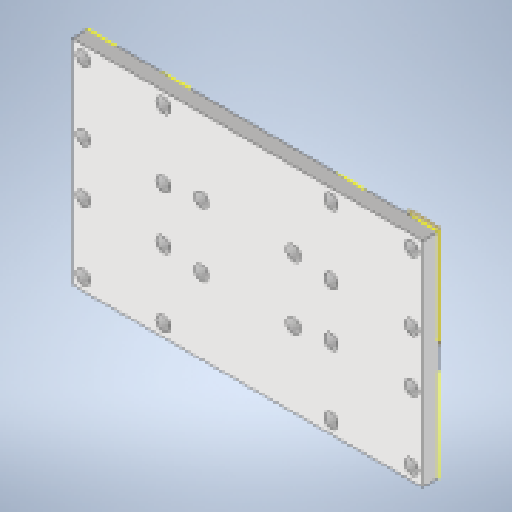
# Autodesk Inventor part: X_PLATE
Saved by Autodesk Inventor 2025.2 (Build 292293000, 293)
## iProperties
Created: 2026-02-06
Part Number: X_PLATE
Material: Generic
Document SubType Name: Modeling
Designer: composite
Density: 1 g/cm^3
Appearance: Default
Author: composite
Autodesk Inventor part; units mm, degrees
ref_plane "YZ Plane" through (0, 0, 0) normal (1, 0, 0) x (0, 1, 0)
ref_plane "XZ Plane" through (0, 0, 0) normal (0, 1, 0) x (-1, 0, 0)
ref_plane "XY Plane" through (0, 0, 0) normal (0, 0, 1) x (1, 0, 0)
ref_plane "Work Plane1" through (4.9275, 0, 0) normal (0, 0, 1) x (1, 0, 0)
sketch "Sketch1" plane through (4.9275, 0, 0) normal (0, 0, 1) x (1, 0, 0)
  line L0 (-4.9275, 35.6) -> (-15.6775, 35.6) projected
  line L1 (-15.6775, 35.6) -> (-15.6775, 0.4) projected
  line L2 (-15.6775, 0.4) -> (-4.9275, 0.4) projected
  line L3 (-4.9275, 35.6) -> (-4.9275, 0.4) projected
  circle A0 centre (-9.1775, 5) radius 2.5 projected
  circle A1 centre (-9.1775, 31) radius 2.5 projected
  line L4 (-4.9275, -10.4) -> (-15.6775, -10.4) projected
  line L5 (-15.6775, -10.4) -> (-15.6775, -45.6) projected
  line L6 (-15.6775, -45.6) -> (-4.9275, -45.6) projected
  line L7 (-4.9275, -10.4) -> (-4.9275, -45.6) projected
  circle A2 centre (-9.1775, -41) radius 2.5 projected
  circle A3 centre (-9.1775, -15) radius 2.5 projected
  line L8 (-33.1775, -10.4) -> (-43.9275, -10.4) projected
  line L9 (-43.9275, -10.4) -> (-43.9275, -45.6) projected
  line L10 (-43.9275, -45.6) -> (-33.1775, -45.6) projected
  line L11 (-33.1775, -45.6) -> (-33.1775, -10.4) projected
  circle A4 centre (-39.6775, -41) radius 2.5 projected
  circle A5 centre (-39.6775, -15) radius 2.5 projected
  line L12 (-33.1775, 35.6) -> (-43.9275, 35.6) projected
  line L13 (-43.9275, 35.6) -> (-43.9275, 0.4) projected
  line L14 (-43.9275, 0.4) -> (-33.1775, 0.4) projected
  line L15 (-33.1775, 0.4) -> (-33.1775, 35.6) projected
  circle A6 centre (-39.6775, 5) radius 2.5 projected
  circle A7 centre (-39.6775, 31) radius 2.5 projected
  circle A8 centre (-89.1275, 7) radius 2.5 projected
  circle A9 centre (-54.1275, -17) radius 2.5 projected
  circle A10 centre (-89.1275, -17) radius 2.5 projected
  circle A11 centre (-54.1275, 7) radius 2.5 projected
  line L16 (-46.6275, 13) -> (-96.6275, 13) projected
  line L17 (-96.6275, 13) -> (-96.6275, -23) projected
  line L18 (-46.6275, -23) -> (-96.6275, -23) projected
  line L19 (-46.6275, 13) -> (-46.6275, -23) projected
  line L20 (-110.0775, 0.4) -> (-99.3275, 0.4) projected
  line L21 (-99.3275, 0.4) -> (-99.3275, 35.6) projected
  line L22 (-99.3275, 35.6) -> (-110.0775, 35.6) projected
  line L23 (-110.0775, 35.6) -> (-110.0775, 0.4) projected
  circle A12 centre (-103.5775, 31) radius 2.5 projected
  circle A13 centre (-103.5775, 5) radius 2.5 projected
  line L24 (-138.3275, 0.4) -> (-127.5775, 0.4) projected
  line L25 (-127.5775, 0.4) -> (-127.5775, 35.6) projected
  line L26 (-127.5775, 35.6) -> (-138.3275, 35.6) projected
  line L27 (-138.3275, 0.4) -> (-138.3275, 35.6) projected
  circle A14 centre (-134.0775, 31) radius 2.5 projected
  circle A15 centre (-134.0775, 5) radius 2.5 projected
  line L28 (-138.3275, -45.6) -> (-127.5775, -45.6) projected
  line L29 (-127.5775, -45.6) -> (-127.5775, -10.4) projected
  line L30 (-127.5775, -10.4) -> (-138.3275, -10.4) projected
  line L31 (-138.3275, -45.6) -> (-138.3275, -10.4) projected
  circle A16 centre (-134.0775, -15) radius 2.5 projected
  circle A17 centre (-134.0775, -41) radius 2.5 projected
  line L32 (-110.0775, -45.6) -> (-99.3275, -45.6) projected
  line L33 (-99.3275, -45.6) -> (-99.3275, -10.4) projected
  line L34 (-99.3275, -10.4) -> (-110.0775, -10.4) projected
  line L35 (-110.0775, -10.4) -> (-110.0775, -45.6) projected
  circle A18 centre (-103.5775, -15) radius 2.5 projected
  circle A19 centre (-103.5775, -41) radius 2.5 projected
  point P0 (-4.9275, 0)
ref_plane "Work Plane2" through (4.9275, 0, 0) normal (0, 0, 1) x (1, 0, 0)
sketch "Sketch2" plane through (4.9275, 0, 0) normal (0, 0, 1) x (1, 0, 0)
  line L0 (-4.9275, 35.6) -> (-4.9275, 0.4) projected
  line L1 (-4.9275, 35.6) -> (-15.6775, 35.6) projected
  line L2 (-138.3275, -45.6) -> (-127.5775, -45.6) projected
  line L3 (-138.3275, -45.6) -> (-138.3275, -10.4) projected
  line L4 (-4.9275, 35.6) -> (-138.3275, 35.6)
  line L5 (-138.3275, 35.6) -> (-138.3275, -45.6)
  line L6 (-138.3275, -45.6) -> (-4.9275, -45.6)
  line L7 (-4.9275, -45.6) -> (-4.9275, 35.6)
  circle A0 centre (-9.1775, 31) radius 2.7
  circle A1 centre (-9.1775, 5) radius 2.7
  circle A2 centre (-9.1775, -15) radius 2.7
  circle A3 centre (-9.1775, -41) radius 2.7
  circle A4 centre (-39.6775, -41) radius 2.7
  circle A5 centre (-39.6775, -15) radius 2.7
  circle A6 centre (-39.6775, 5) radius 2.7
  circle A7 centre (-39.6775, 31) radius 2.7
  circle A8 centre (-103.5775, 31) radius 2.7
  circle A9 centre (-103.5775, 5) radius 2.7
  circle A10 centre (-103.5775, -15) radius 2.7
  circle A11 centre (-103.5775, -41) radius 2.7
  circle A12 centre (-134.0775, -41) radius 2.7
  circle A13 centre (-134.0775, -15) radius 2.7
  circle A14 centre (-134.0775, 5) radius 2.7
  circle A15 centre (-134.0775, 31) radius 2.7
  circle A16 centre (-54.1275, 7) radius 2.7
  circle A17 centre (-54.1275, -17) radius 2.7
  circle A18 centre (-89.1275, -17) radius 2.7
  circle A19 centre (-89.1275, 7) radius 2.7
  point P0 (-4.9275, 0)
  dimension "d0" = 5.4
  constraints: 20 centre point, 20 coincident, 19 equal radius, 8 end point, 2 parallel, 1 horizontal, 1 perpendicular
  measures "d0" diameter of A0
extrude "Extrusion1" add sketch "Sketch2" along normal blind 6
body "Solid1"
